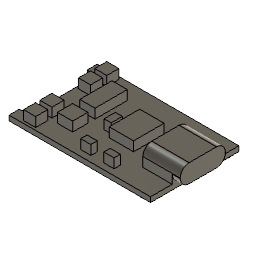
4056 Battery Charger (Autodesk Fusion 360 design; units mm, degrees)
Autodesk Fusion 360 part; units mm, degrees
note: some values were not read from the file. Set by a fixed rule: which sketch regions a step uses.
sketch "Sketch1" plane through (0, 0, 0) normal (0, 0, 1) x (1, 0, 0)
  line L0 (0, 0) -> (27.85, 0)
  line L1 (27.85, 0) -> (27.85, 17.4)
  line L2 (27.85, 17.4) -> (0, 17.4)
  line L3 (1.8536, 13.55) -> (1.8536, 3.85)
  line L4 (0, 17.4) -> (0, 15.4)
  line L5 (0, 0) -> (0, 2)
  line L6 (0, 15.4) -> (0.0036, 15.4)
  line L7 (0, 2) -> (0.0036, 2)
  arc A0 (1.8536, 13.55) -> (0.0036, 15.4) centre (0.0036, 13.55) ccw
  arc A1 (0.0036, 2) -> (1.8536, 3.85) centre (0.0036, 3.85) ccw
  dimension "d2" = 27.85
  dimension "d27" = 17.4
  dimension "d28" = 2
  dimension "d29" = 2
  dimension "d32" = 1.85
  constraint horizontal L0
  constraint vertical L1
  constraint horizontal L2
  constraint coincident L0.start L5.start
  constraint perpendicular L2 L4
  constraint perpendicular L0 L5
  constraint vertical L3
  constraint perpendicular L3 L6
  constraint perpendicular L3 L7
  constraint tangent L6 A0
  constraint tangent L3 A0
  constraint tangent L7 A1
  constraint tangent L3 A1
  constraint equal A0 A1
  measures "d2" distance of L0.start L0.end
  measures "d27" distance of L0.end L1.end
  measures "d28" distance of L2.end L4.end
  measures "d29" distance of L0.start L5.end
  measures "d32" radius of A0
extrude "Extrude1" add sketch "Sketch1" along normal blind 1
sketch "Sketch2" plane through (0, 0, 1) normal (0, 0, 1) x (-1, 0, 0)
  line L0 (0, 0) -> (-27.85, 0)
  line L1 (-27.85, 0) -> (-27.85, -17.4)
  line L2 (-27.85, -17.4) -> (0, -17.4)
  line L3 (-6.16, -14.12) -> (-9.16, -14.12)
  line L4 (-9.16, -14.12) -> (-9.16, -7.77)
  line L5 (-9.16, -7.77) -> (-6.16, -7.77)
  line L6 (-6.16, -7.77) -> (-6.16, -14.12)
  line L7 (-13.7136, -12) -> (-18.5136, -12)
  line L8 (-18.5136, -12) -> (-18.5136, -6)
  line L9 (-18.5136, -6) -> (-13.7136, -6)
  line L10 (-13.7136, -6) -> (-13.7136, -12)
  line L11 (-6.16, -6.37) -> (-9.16, -6.37)
  line L12 (-9.16, -6.37) -> (-9.16, -3.37)
  line L13 (-9.16, -3.37) -> (-6.16, -3.37)
  line L14 (-6.16, -3.37) -> (-6.16, -6.37)
  line L15 (-11.8536, -9.06) -> (-13.2536, -9.06)
  line L16 (-13.2536, -9.06) -> (-13.2536, -6.86)
  line L17 (-13.2536, -6.86) -> (-11.8536, -6.86)
  line L18 (-11.8536, -6.86) -> (-11.8536, -9.06)
  line L19 (-12.94, -2.43) -> (-14.94, -2.43)
  line L20 (-14.94, -2.43) -> (-14.94, -1.18)
  line L21 (-14.94, -1.18) -> (-12.94, -1.18)
  line L22 (-12.94, -1.18) -> (-12.94, -2.43)
  line L23 (-17.49, -2.43) -> (-19.49, -2.43)
  line L24 (-19.49, -2.43) -> (-19.49, -1.18)
  line L25 (-19.49, -1.18) -> (-17.49, -1.18)
  line L26 (-17.49, -1.18) -> (-17.49, -2.43)
  line L27 (-2.3536, -16.9) -> (-4.7536, -16.9)
  line L28 (-4.7536, -16.9) -> (-4.7536, -14.5)
  line L29 (-4.7536, -14.5) -> (-2.3536, -14.5)
  line L30 (-2.3536, -14.5) -> (-2.3536, -16.9)
  line L31 (-2.3536, -13.7) -> (-4.7536, -13.7)
  line L32 (-4.7536, -13.7) -> (-4.7536, -11.3)
  line L33 (-4.7536, -11.3) -> (-2.3536, -11.3)
  line L34 (-2.3536, -11.3) -> (-2.3536, -13.7)
  line L35 (-2.3536, -2.9) -> (-4.7536, -2.9)
  line L36 (-4.7536, -2.9) -> (-4.7536, -0.5)
  line L37 (-4.7536, -0.5) -> (-2.3536, -0.5)
  line L38 (-2.3536, -0.5) -> (-2.3536, -2.9)
  line L39 (-2.3536, -6.1) -> (-4.7536, -6.1)
  line L40 (-4.7536, -6.1) -> (-4.7536, -3.7)
  line L41 (-4.7536, -3.7) -> (-2.3536, -3.7)
  line L42 (-2.3536, -3.7) -> (-2.3536, -6.1)
  line L43 (0, -17.4) -> (0, -15.4)
  line L44 (0, -15.4) -> (-0.0036, -15.4)
  arc A0 (-1.8536, -13.55) -> (-0.0036, -15.4) centre (-0.0036, -13.55) ccw
  line L45 (-1.8536, -13.55) -> (-1.8536, -3.85)
  arc A1 (-0.0036, -2) -> (-1.8536, -3.85) centre (-0.0036, -3.85) ccw
  line L46 (-0.0036, -2) -> (0, -2)
  line L47 (0, -2) -> (0, 0)
  dimension "d5" = 4.8
  dimension "d6" = 6
  dimension "d7" = 1.4
  dimension "d8" = 2.2
  dimension "d9" = 3
  dimension "d10" = 6.35
  dimension "d11" = 3
  dimension "d12" = 3
  dimension "d13" = 2
  dimension "d14" = 1.25
  dimension "d15" = 2
  dimension "d16" = 1.25
  dimension "d17" = 2.4
  dimension "d18" = 2.4
  dimension "d19" = 2.4
  dimension "d20" = 2.4
  dimension "d21" = 2.4
  dimension "d22" = 2.4
  dimension "d23" = 2.4
  dimension "d24" = 2.4
  dimension "d25" = 3.28
  dimension "d33" = 0.5
  dimension "d34" = 0.5
  dimension "d35" = 0.5
  dimension "d36" = 0.8
  dimension "d37" = 0.8
  dimension "d38" = 6.16
  dimension "d39" = 1.4
  dimension "d40" = 6.86
  dimension "d41" = 10
  dimension "d42" = 11.86
  dimension "d43" = 5.4
  dimension "d44" = 1.18
  dimension "d45" = 2.55
  dimension "d46" = 8.36
  constraint horizontal L3
  constraint vertical L4
  constraint horizontal L5
  constraint vertical L6
  constraint horizontal L7
  constraint vertical L8
  constraint horizontal L9
  constraint vertical L10
  constraint horizontal L11
  constraint vertical L12
  constraint horizontal L13
  constraint vertical L14
  constraint horizontal L15
  constraint vertical L16
  constraint horizontal L17
  constraint vertical L18
  constraint horizontal L19
  constraint vertical L20
  constraint horizontal L21
  constraint vertical L22
  constraint horizontal L23
  constraint vertical L24
  constraint horizontal L25
  constraint vertical L26
  constraint horizontal L27
  constraint vertical L28
  constraint horizontal L29
  constraint vertical L30
  constraint horizontal L31
  constraint vertical L32
  constraint horizontal L33
  constraint vertical L34
  constraint horizontal L35
  constraint vertical L36
  constraint horizontal L37
  constraint vertical L38
  constraint horizontal L39
  constraint vertical L40
  constraint horizontal L41
  constraint vertical L42
  constraint collinear L38 L42
  constraint collinear L34 L42
  constraint collinear L30 L34
  constraint collinear L6 L14
  constraint collinear L21 L25
  measures "d5" distance of L7.start L7.end
  measures "d6" distance of L7.start L9.end
  measures "d7" distance of L15.start L15.end
  measures "d8" distance of L15.start L17.end
  measures "d9" distance of L3.start L3.end
  measures "d10" distance of L3.start L5.end
  measures "d11" distance of L11.start L11.end
  measures "d12" distance of L11.start L13.end
  measures "d13" distance of L19.start L19.end
  measures "d14" distance of L19.start L21.end
  measures "d15" distance of L23.start L23.end
  measures "d16" distance of L23.start L25.end
  measures "d17" distance of L35.start L35.end
  measures "d18" distance of L35.start L37.end
  measures "d19" distance of L40.end L41.end
  measures "d20" distance of L39.start L41.end
  measures "d21" distance of L31.start L31.end
  measures "d22" distance of L31.start L33.end
  measures "d23" distance of L27.start L27.end
  measures "d24" distance of L27.start L29.end
  measures "d25" distance of L2 L3
  measures "d33" distance of L2 L27
  measures "d34" distance of L0 L37
  measures "d35" distance of L38 L45
  measures "d36" distance of L35 L41
  measures "d37" distance of L29 L31
  measures "d38" distance of L6 L43
  measures "d39" distance of L5 L11
  measures "d40" distance of L0 L17
  measures "d41" distance of L18 L45
  measures "d42" distance of L10 L45
  measures "d43" distance of L2 L7
  measures "d44" distance of L0 L21
  measures "d45" distance of L20 L26
  measures "d46" distance of L1 L24
extrude "Extrude2" add sketch "Sketch2" along normal blind 1.86 contours L3 L4 L5 L6 | L7 L8 L9 L10 | L11 L12 L13 L14 | L15 L16 L17 L18 | L19 L20 L21 L22 | L23 L24 L25 L26 | L27 L28 L29 L30 | L31 L32 L33 L34 | L35 L36 L37 L38 | L39 L40 L41 L42
sketch "Sketch3" plane through (0, 0, 1) normal (0, 0, 1) x (-1, 0, 0)
  line L0 (-17.49, -1.18) -> (-17.49, -2.43)
  line L1 (-17.49, -2.43) -> (-19.49, -2.43)
  line L2 (-19.49, -2.43) -> (-19.49, -1.18)
  line L3 (-19.49, -1.18) -> (-17.49, -1.18)
  line L4 (-6.16, -3.37) -> (-6.16, -6.37)
  line L5 (-6.16, -6.37) -> (-9.16, -6.37)
  line L6 (-9.16, -6.37) -> (-9.16, -3.37)
  line L7 (-9.16, -3.37) -> (-6.16, -3.37)
  line L8 (-2.3536, -3.7) -> (-2.3536, -6.1)
  line L9 (-2.3536, -6.1) -> (-4.7536, -6.1)
  line L10 (-4.7536, -6.1) -> (-4.7536, -3.7)
  line L11 (-4.7536, -3.7) -> (-2.3536, -3.7)
  line L12 (-2.3536, -11.3) -> (-2.3536, -13.7)
  line L13 (-2.3536, -13.7) -> (-4.7536, -13.7)
  line L14 (-4.7536, -13.7) -> (-4.7536, -11.3)
  line L15 (-4.7536, -11.3) -> (-2.3536, -11.3)
  line L16 (-11.8536, -6.86) -> (-11.8536, -9.06)
  line L17 (-11.8536, -9.06) -> (-13.2536, -9.06)
  line L18 (-13.2536, -9.06) -> (-13.2536, -6.86)
  line L19 (-13.2536, -6.86) -> (-11.8536, -6.86)
  line L20 (-12.94, -1.18) -> (-12.94, -2.43)
  line L21 (-12.94, -2.43) -> (-14.94, -2.43)
  line L22 (-14.94, -2.43) -> (-14.94, -1.18)
  line L23 (-14.94, -1.18) -> (-12.94, -1.18)
  line L24 (-6.16, -7.77) -> (-6.16, -14.12)
  line L25 (-6.16, -14.12) -> (-9.16, -14.12)
  line L26 (-9.16, -14.12) -> (-9.16, -7.77)
  line L27 (-9.16, -7.77) -> (-6.16, -7.77)
  line L28 (-2.3536, -0.5) -> (-2.3536, -2.9)
  line L29 (-2.3536, -2.9) -> (-4.7536, -2.9)
  line L30 (-4.7536, -2.9) -> (-4.7536, -0.5)
  line L31 (-4.7536, -0.5) -> (-2.3536, -0.5)
  line L32 (-2.3536, -14.5) -> (-2.3536, -16.9)
  line L33 (-2.3536, -16.9) -> (-4.7536, -16.9)
  line L34 (-4.7536, -16.9) -> (-4.7536, -14.5)
  line L35 (-4.7536, -14.5) -> (-2.3536, -14.5)
  line L36 (-13.7136, -6) -> (-13.7136, -12)
  line L37 (-13.7136, -12) -> (-18.5136, -12)
  line L38 (-18.5136, -12) -> (-18.5136, -6)
  line L39 (-18.5136, -6) -> (-13.7136, -6)
  line L40 (0, 0) -> (-27.85, 0)
  line L41 (-27.85, 0) -> (-27.85, -17.4)
  line L42 (-27.85, -17.4) -> (0, -17.4)
  line L43 (0, -17.4) -> (0, -15.4)
  line L44 (0, -15.4) -> (-0.0036, -15.4)
  arc A0 (-1.8536, -13.55) -> (-0.0036, -15.4) centre (-0.0036, -13.55) ccw
  line L45 (-1.8536, -13.55) -> (-1.8536, -3.85)
  arc A1 (-0.0036, -2) -> (-1.8536, -3.85) centre (-0.0036, -3.85) ccw
  line L46 (-0.0036, -2) -> (0, -2)
  line L47 (0, -2) -> (0, 0)
  line L48 (-22.08, -13.14) -> (-29.43, -13.14)
  line L49 (-29.43, -13.14) -> (-29.43, -4.26)
  line L50 (-29.43, -4.26) -> (-22.08, -4.26)
  line L51 (-22.08, -4.26) -> (-22.08, -13.14)
  dimension "d49" = 7.35
  dimension "d50" = 8.88
  dimension "d51" = 4.26
  dimension "d52" = 1.58
  constraint horizontal L48
  constraint vertical L49
  constraint horizontal L50
  constraint vertical L51
  measures "d49" distance of L48.start L48.end
  measures "d50" distance of L48.start L50.end
  measures "d51" distance of L40 L50
  measures "d52" distance of L41 L49
extrude "Extrude3" add sketch "Sketch3" along normal blind 3.6 contours L41 L48 L50 L51 | L41 L48 L49 L50
fillet "Fillet1" radius 1.75 4 edges at (28.64, 13.14, 1) (25.755, 13.14, 4.6) (25.755, 4.26, 4.6) (28.64, 4.26, 1)
sketch "Sketch4" plane through (0, 0, 0) normal (0, 0, -1) x (1, 0, 0)
  line L0 (27.85, 0) -> (0, 0)
  line L1 (0, 0) -> (0, -2)
  line L2 (0, -2) -> (0.0036, -2)
  arc A0 (1.8536, -3.85) -> (0.0036, -2) centre (0.0036, -3.85) ccw
  line L3 (1.8536, -3.85) -> (1.8536, -13.55)
  arc A1 (0.0036, -15.4) -> (1.8536, -13.55) centre (0.0036, -13.55) ccw
  line L4 (0.0036, -15.4) -> (0, -15.4)
  line L5 (0, -15.4) -> (0, -17.4)
  line L6 (0, -17.4) -> (27.85, -17.4)
  line L7 (27.85, -17.4) -> (27.85, 0)
  line L8 (2.3536, -0.5) -> (4.7536, -0.5)
  line L9 (4.7536, -0.5) -> (4.7536, -2.9)
  line L10 (4.7536, -2.9) -> (2.3536, -2.9)
  line L11 (2.3536, -2.9) -> (2.3536, -0.5)
  line L12 (27.35, -16.4) -> (24.95, -16.4)
  line L13 (24.95, -16.4) -> (24.95, -14)
  line L14 (24.95, -14) -> (27.35, -14)
  line L15 (27.35, -14) -> (27.35, -16.4)
  line L16 (4.7536, -5.9) -> (2.3536, -5.9)
  line L17 (2.3536, -5.9) -> (2.3536, -3.5)
  line L18 (2.3536, -3.5) -> (4.7536, -3.5)
  line L19 (4.7536, -3.5) -> (4.7536, -5.9)
  line L20 (4.7536, -13.4) -> (2.3536, -13.4)
  line L21 (2.3536, -13.4) -> (2.3536, -11)
  line L22 (2.3536, -11) -> (4.7536, -11)
  line L23 (4.7536, -11) -> (4.7536, -13.4)
  line L24 (4.7536, -16.4) -> (2.3536, -16.4)
  line L25 (2.3536, -16.4) -> (2.3536, -14)
  line L26 (2.3536, -14) -> (4.7536, -14)
  line L27 (4.7536, -14) -> (4.7536, -16.4)
  line L28 (27.35, -2.9) -> (24.95, -2.9)
  line L29 (24.95, -2.9) -> (24.95, -0.5)
  line L30 (24.95, -0.5) -> (27.35, -0.5)
  line L31 (27.35, -0.5) -> (27.35, -2.9)
  line L32 (4.7536, -0.5) -> (2.3536, -0.5)
  line L33 (2.3536, -0.5) -> (2.3536, -2.9)
  dimension "d57" = 2.4
  dimension "d58" = 2.4
  dimension "d59" = 2.4
  dimension "d60" = 2.4
  dimension "d61" = 2.4
  dimension "d62" = 2.4
  dimension "d63" = 2.4
  dimension "d64" = 2.4
  dimension "d65" = 2.4
  dimension "d66" = 2.4
  dimension "d67" = 2.4
  dimension "d68" = 2.4
  dimension "d69" = 0.5
  constraint horizontal L8
  constraint vertical L9
  constraint horizontal L10
  constraint vertical L11
  constraint horizontal L14
  constraint vertical L15
  constraint horizontal L12
  constraint vertical L13
  constraint horizontal L18
  constraint vertical L19
  constraint horizontal L16
  constraint vertical L17
  constraint horizontal L22
  constraint vertical L23
  constraint horizontal L20
  constraint vertical L21
  constraint horizontal L26
  constraint vertical L27
  constraint horizontal L24
  constraint vertical L25
  constraint horizontal L30
  constraint vertical L31
  constraint horizontal L28
  constraint vertical L29
  constraint collinear L8 L30
  constraint collinear L15 L31
  constraint collinear L12 L24
  constraint collinear L21 L25
  constraint collinear L17 L21
  constraint collinear L11 L17
  constraint collinear L8 L32
  constraint collinear L11 L33
  measures "d57" distance of L8.start L8.end
  measures "d58" distance of L8.start L10.end
  measures "d59" distance of L13.end L14.end
  measures "d60" distance of L13.end L12.end
  measures "d61" distance of L17.end L18.end
  measures "d62" distance of L17.end L16.end
  measures "d63" distance of L21.end L22.end
  measures "d64" distance of L21.end L20.end
  measures "d65" distance of L25.end L26.end
  measures "d66" distance of L25.end L24.end
  measures "d67" distance of L29.end L30.end
  measures "d68" distance of L29.end L28.end
  measures "d69" distance of L7 L31
extrude "Extrude4" add sketch "Sketch4" along normal blind 1 contours L8 L9 L10 L11 L32 L33 | L12 L13 L14 L15 | L16 L17 L18 L19 | L20 L21 L22 L23 | L24 L25 L26 L27 | L28 L29 L30 L31
fillet "Fillet2" radius 0.75 6 faces at (3.1536, 1.3, -1) (3.9536, 5.1, -1) (3.9536, 12.6, -1) (3.9536, 15.6, -1) (25.75, 15.6, -1) (25.75, 2.1, -1)
equation "d15 = d13"
equation "d16 = d14"
equation "d18 = d17"
equation "d19 = d17"
equation "d20 = d17"
equation "d21 = d17"
equation "d22 = d17"
equation "d23 = d17"
equation "d24 = d17"
equation "d51 = ( d27 - d50 ) / 2"
